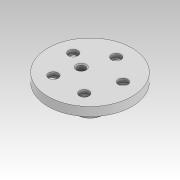
# Autodesk Inventor part: Flywheel
Saved by Autodesk Inventor 2020 (Build 240168000, 168)
## iProperties
Created: 2021-10-30
Part Number: Flywheel
Material: Generic
Document SubType Name: Modeling
Designer: DDeGo
Density: 1 g/cm^3
Appearance: Default
Author: DDeGo
Autodesk Inventor part; units mm, degrees
ref_plane "YZ Plane" through (0, 0, 0) normal (1, 0, 0) x (0, 1, 0)
ref_plane "XZ Plane" through (0, 0, 0) normal (0, 1, 0) x (-1, 0, 0)
ref_plane "XY Plane" through (0, 0, 0) normal (0, 0, 1) x (1, 0, 0)
sketch "Sketch1" plane through (0, 0, 0) normal (0, 0, 1) x (1, 0, 0)
  line L0 (0, 8.8) -> (0, 0)
  line L1 (0, 0) -> (1, 0)
  line L2 (1, 0) -> (1, 8.8) construction
  line L3 (1, 8.8) -> (0, 8.8)
  line L4 (1, 8.8) -> (12, 8.8)
  line L5 (4.45, 3.8) -> (3.95, 3.8)
  line L6 (3.95, 3.8) -> (3.95, 0)
  line L7 (3.95, 0) -> (1, 0)
  line L8 (12, 8.8) -> (12, 6.3)
  line L9 (12, 6.3) -> (4.95, 6.3)
  line L10 (4.95, 6.3) -> (4.45, 3.8)
  dimension "d0" = 3.95
  dimension "d1" = 1
  dimension "d3" = 0.5
  dimension "d4" = 3.8
  dimension "d10" = 12
  dimension "d11" = 2.5
  dimension "d35" = 2.5
  dimension "d43" = 0.5
  constraints: 22 end point, 6 perpendicular, 2 vertical, 1 horizontal
  measures "d0" distance between parallel lines of L0 L6
  measures "d1" distance between parallel lines of L0 L2
  measures "d3" distance of L5.start L5.end
  measures "d4" distance of L5.end L6.end
  measures "d10" distance between parallel lines of L0 L8
  measures "d11" distance of L4.end L8.end
  measures "d35" distance between parallel lines of L5 L9
  measures "d43" horizontal distance of L5.start L9.end
revolve "Revolution1" add sketch "Sketch1" angle 360 about axis through (0, 8.8, 0) along (0, -1, 0)
sketch "Sketch2" plane through (0, 8.8, 0) normal (0, 1, 0) x (1, 0, 0)
  line L0 (0, 0) -> (0, 7.5) construction
  circle A0 centre (0, 7.5) radius 1.35
  line L1 (0, 0) -> (-7.1329, 2.3176) construction
  circle A1 centre (-7.1329, 2.3176) radius 1.35
  line L2 (0, 0) -> (-4.4084, -6.0676) construction
  circle A2 centre (-4.4084, -6.0676) radius 1.35
  line L3 (0, 0) -> (4.4084, -6.0676) construction
  circle A3 centre (4.4084, -6.0676) radius 1.35
  line L4 (0, 0) -> (7.1329, 2.3176) construction
  circle A4 centre (7.1329, 2.3176) radius 1.35
  dimension "d12" = 7.5
  dimension "d13" = 2.7
  dimension "d16" = 360
  constraints: 10 end point, 7 coincident, 5 centre point, 1 vertical, 24 other
  measures "d12" distance of L0.start L0.end
  measures "d13" diameter of A0
extrude "Extrusion1" cut sketch "Sketch2" against normal up to surface (2.5 mm away)
sketch "Sketch3" plane through (0, 6.3, 0) normal (0, -1, 0) x (1, 0, 0)
  circle A0 centre (0, -7.5) radius 1.35 construction
  line L0 (-2.9445, -7.5) -> (-1.4722, -4.95)
  line L1 (-1.4722, -4.95) -> (1.4722, -4.95)
  line L2 (1.4722, -4.95) -> (2.9445, -7.5)
  line L3 (2.9445, -7.5) -> (1.4722, -10.05)
  line L4 (1.4722, -10.05) -> (-1.4722, -10.05)
  line L5 (-1.4722, -10.05) -> (-2.9445, -7.5)
  line L6 (6.223, -5.118) -> (4.2528, -2.9298)
  line L7 (4.2528, -2.9298) -> (5.1627, -0.1294)
  line L8 (5.1627, -0.1294) -> (8.0428, 0.4827)
  line L9 (8.0428, 0.4827) -> (10.0131, -1.7054)
  line L10 (10.0131, -1.7054) -> (9.1032, -4.5058)
  line L11 (9.1032, -4.5058) -> (6.223, -5.118)
  line L12 (6.7905, 4.3369) -> (4.1006, 3.1393)
  line L13 (4.1006, 3.1393) -> (1.7185, 4.87)
  line L14 (1.7185, 4.87) -> (2.0262, 7.7984)
  line L15 (2.0262, 7.7984) -> (4.7162, 8.996)
  line L16 (4.7162, 8.996) -> (7.0983, 7.2653)
  line L17 (7.0983, 7.2653) -> (6.7905, 4.3369)
  line L18 (-2.0262, 7.7984) -> (-1.7185, 4.87)
  line L19 (-1.7185, 4.87) -> (-4.1006, 3.1393)
  line L20 (-4.1006, 3.1393) -> (-6.7905, 4.3369)
  line L21 (-6.7905, 4.3369) -> (-7.0983, 7.2653)
  line L22 (-7.0983, 7.2653) -> (-4.7162, 8.996)
  line L23 (-4.7162, 8.996) -> (-2.0262, 7.7984)
  line L24 (-8.0428, 0.4827) -> (-5.1627, -0.1294)
  line L25 (-5.1627, -0.1294) -> (-4.2528, -2.9298)
  line L26 (-4.2528, -2.9298) -> (-6.223, -5.118)
  line L27 (-6.223, -5.118) -> (-9.1032, -4.5058)
  line L28 (-9.1032, -4.5058) -> (-10.0131, -1.7054)
  line L29 (-10.0131, -1.7054) -> (-8.0428, 0.4827)
  point P0 (0, 0)
  point P1 (0, -7.5)
  point P2 (7.1329, -2.3176)
  point P3 (7.1329, -2.3176)
  point P4 (4.4084, 6.0676)
  point P5 (4.4084, 6.0676)
  point P6 (-4.4084, 6.0676)
  point P7 (-4.4084, 6.0676)
  point P8 (-7.1329, -2.3176)
  point P9 (-7.1329, -2.3176)
  point P10 (5.95, 0)
  point P11 (5.95, 0)
  dimension "d20" = 5.1
  dimension "d23" = 360
  constraints: 60 end point, 5 coincident, 1 horizontal, 85 other
  measures "d20" distance between parallel lines of L1 L4
extrude "Extrusion2" cut sketch "Sketch3" against normal blind 1.5
sketch "Sketch5" plane through (0, 0, 0) normal (0, -1, 0) x (1, 0, 0)
  line L0 (0, 0) -> (-2.5, 0) construction
  circle A0 centre (-2.5, 0) radius 1.125
  dimension "d36" = 2.5
  dimension "d37" = 2.25
  constraints: 2 end point, 1 centre point, 1 coincident, 1 horizontal
  measures "d36" distance of L0.start L0.end
  measures "d37" diameter of A0
extrude "Extrusion4" cut sketch "Sketch5" against normal through all
chamfer "Chamfer3" distance 0.3 angle 45 2 edges at (-3.625, 0, 0) (-3.625, 8.8, 0)
chamfer "Chamfer4" distance 0.3 angle 45 1 edges at (-3.95, 0, 0)
sketch "Sketch6" plane through (0, 0, 0) normal (0, -1, 0) x (1, 0, 0)
  line L0 (-5.4879, 0.4) -> (-2.4549, 0.4)
  line L1 (-2.4549, 0.4) -> (-2.4549, -0.4)
  line L2 (-2.4549, -0.4) -> (-5.4879, -0.4)
  line L3 (-5.4879, -0.4) -> (-5.4879, 0.4)
  point P0 (0, 0)
  dimension "d47" = 0.4
  dimension "d48" = 0.4
  constraints: 8 end point, 2 parallel, 1 horizontal, 1 perpendicular
  measures "d47" distance from line of point (0, 0) L2
  measures "d48" distance from line of point (0, 0) L0
extrude "Extrusion5" cut sketch "Sketch6" against normal up to surface (3.8 mm away)
fillet "Fillet2" radius 0.35 4 edges at (-3.5515, 2.05, 0.4) (-3.9297, 2.05, 0.4) (-3.9297, 2.05, -0.4) (-3.5515, 2.05, -0.4)
equation "\"d48\" = d47"
body "Solid1"
